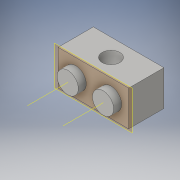
# Autodesk Inventor part: bricks
Saved by Autodesk Inventor 2016 (Build 200138000, 138)
## iProperties
Created: 2018-02-13
Part Number: bricks
Material: Generic
Document SubType Name: Modeling
Designer: sun01147
Density: 1 g/cm^3
Appearance: Default
Author: sun01147
Autodesk Inventor part; units mm, degrees
ref_plane "YZ Plane" through (0, 0, 0) normal (1, 0, 0) x (0, 1, 0)
ref_plane "XZ Plane" through (0, 0, 0) normal (0, 1, 0) x (-1, 0, 0)
sketch "Top" plane through (0, 0, 0) normal (0, 0, 1) x (1, 0, 0)
  line L0 (0, 8) -> (0, 0)
  line L1 (0, 0) -> (16, 0)
  line L2 (16, 0) -> (16, 8)
  line L3 (0, 8) -> (16, 8)
  point P0 (8, 0)
  dimension "d0" = 16
  dimension "d1" = 8
  dimension "d2" = 8
  constraints: 8 end point, 2 perpendicular, 1 midpoint, 1 vertical
  measures "d0" distance of L0.end L1.end
  measures "d1" distance of L0.start L0.end
  measures "d2" distance of L1.end L2.end
extrude "Extrusion5" add sketch "Top" against normal blind 8
sketch "Sketch4" plane through (0, 0, 0) normal (0, 0, 1) x (1, 0, 0)
  line L0 (0, 0) -> (0, 8) projected
  line L1 (16, 8) -> (16, 0) projected
  line L2 (0, 8) -> (16, 8)
  line L3 (16, 8) -> (16, 0)
  line L4 (16, 0) -> (0, 0)
  line L5 (0, 0) -> (0, 8)
  circle A0 centre (4, 4) radius 2.4
  circle A1 centre (12, 4) radius 2.4
  dimension "d29" = 4.8
  dimension "d30" = 4.8
  dimension "d31" = 4
  dimension "d32" = 4
  dimension "d33" = 8
  dimension "d34" = 4
  constraints: 8 end point, 2 centre point, 2 parallel, 1 horizontal, 1 perpendicular
  measures "d29" diameter of A0
  measures "d30" diameter of A1
  measures "d31" distance from line of L0 A0.centre
  measures "d32" distance from line of L4 A0.centre
  measures "d33" distance of A0.centre A1.centre
  measures "d34" distance from line of L4 A1.centre
extrude "Extrusion6" add sketch "Sketch4" along normal blind 1.8 contours A0 | A1
sketch "Sketch5" plane through (0, 0, -8) normal (0, 0, -1) x (-1, 0, 0)
  line L0 (-14.9, 6.9) -> (-1.1, 6.9)
  line L1 (-1.1, 6.9) -> (-1.1, 1.1)
  line L2 (-1.1, 1.1) -> (-14.9, 1.1)
  line L3 (-14.9, 1.1) -> (-14.9, 6.9)
  line L4 (0, 8) -> (-16, 8) projected
  line L5 (-16, 8) -> (-16, 0) projected
  line L6 (-16, 0) -> (0, 0) projected
  line L7 (0, 0) -> (0, 8) projected
  dimension "d37" = 1.1
  dimension "d38" = 1.1
  dimension "d39" = 1.1
  dimension "d40" = 1.1
  constraints: 8 end point, 2 parallel, 1 horizontal, 1 perpendicular
  measures "d37" distance between parallel lines of L4 L0
  measures "d38" distance between parallel lines of L5 L3
  measures "d39" distance between parallel lines of L6 L2
  measures "d40" distance between parallel lines of L7 L1
extrude "Extrusion7" cut sketch "Sketch5" against normal blind 1.2 contours L0 L1 L2 L3
sketch "Sketch6" plane through (0, 0, -6.8) normal (0, 0, -1) x (-1, 0, 0)
  line L0 (-14.9, 1.1) -> (-14.9, 6.9) projected
  line L1 (-14.9, 4.2225) -> (-1.1, 4.2225)
  line L2 (-1.1, 6.9) -> (-1.1, 1.1) projected
  circle A0 centre (-8, 4.2225) radius 2
  line L3 (-16, 8) -> (-16, 0) projected
  line L4 (-1.1, 1.1) -> (-14.9, 1.1) projected
  point P0 (0, 0)
  dimension "d43" = 8
  dimension "d44" = 4
  dimension "d45" = 3.1225
  constraints: 2 end point, 2 point on line, 1 centre point, 1 horizontal, 1 midpoint
  measures "d43" distance from line of L3 A0.centre
  measures "d44" diameter of A0
  measures "d45" distance from line of L4 A0.centre
extrude "Extrusion8" add sketch "Sketch6" along normal blind 1.2 contours A0 L1 | L1 A0
sketch "Sketch8" plane through (0, 8, 0) normal (0, 1, 0) x (1, 0, 0)
  line L0 (16, 0) -> (16, 8) projected
  line L1 (16, 4) -> (0, 4)
  line L2 (0, 0) -> (0, 8) projected
  point P0 (8, 4)
  constraints: 3 midpoint, 2 end point
hole "Hole2" at (8, 8, -4) direction (0, -1, 0) diameter 4 depth 8 tip angle 118
body "Solid2"
